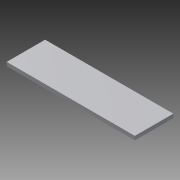
# Autodesk Inventor part: front szuflady 150mm
Saved by Autodesk Inventor 2013 (Build 170138000, 138)
## iProperties
Created: 2014-05-20
Part Number: front szuflady 150mm
Material: Ogólny
Document SubType Name: Modeling
Designer: Piotr
Density: 1 g/cm^3
Author: Piotr
Autodesk Inventor part; units mm, degrees
ref_plane "YZ Plane" through (0, 0, 0) normal (1, 0, 0) x (0, 1, 0)
ref_plane "XZ Plane" through (0, 0, 0) normal (0, 1, 0) x (-1, 0, 0)
ref_plane "XY Plane" through (0, 0, 0) normal (0, 0, 1) x (1, 0, 0)
sketch "Szkic1" plane through (0, 0, 0) normal (0, 0, 1) x (1, 0, 0)
  line L0 (300, -90) -> (-300, -90)
  line L1 (-300, -90) -> (-300, 90)
  line L2 (-300, 90) -> (300, 90)
  line L3 (300, 90) -> (300, -90)
  line L4 (300, -90) -> (-300, 90) construction
  line L5 (-300, -90) -> (300, 90) construction
  line L6 (0, 0) -> (0, 28) construction
  line L7 (257.5, 60) -> (-257.5, 60) construction
  line L8 (-257.5, 60) -> (-257.5, -4) construction
  line L9 (-257.5, -4) -> (257.5, -4) construction
  line L10 (257.5, -4) -> (257.5, 60) construction
  line L11 (257.5, 60) -> (-257.5, -4) construction
  line L12 (-257.5, 60) -> (257.5, -4) construction
  dimension "d0" = 600
  dimension "d2" = 180
  dimension "d3" = 515
  dimension "d4" = 64
  dimension "d5" = 30
  constraints: 26 end point, 5 parallel, 4 coincident, 4 midpoint, 2 horizontal, 2 perpendicular
  measures "d0" distance of L1.end L2.end
  measures "d2" distance of L2.end L0.start
  measures "d3" distance of L9.end L8.end
  measures "d4" distance of L8.end L7.end
  measures "d5" distance between parallel lines of L2 L7
extrude "Wyciągnięcie proste1" add sketch "Szkic1" along normal blind 18
hole "Otwór1" at (-257.5, 60, 0) at (-257.5, -4, 0) at (257.5, 60, 0) at (257.5, -4, 0) direction (0, 0, 1) diameter 3 depth 8 tip angle 118
